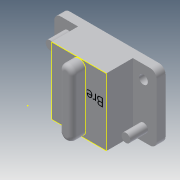
# Autodesk Inventor part: circuit breaker
Saved by Autodesk Inventor 2014 (Build 180170000, 170)
## iProperties
Created: 2016-01-13
Part Number: circuit breaker
Material: Generic
Document SubType Name: Modeling
Designer: Paul
Density: 1 g/cm^3
Appearance: Default
Author: Paul
Autodesk Inventor part; units mm, degrees
ref_plane "YZ Plane" through (0, 0, 0) normal (1, 0, 0) x (0, 1, 0)
ref_plane "XZ Plane" through (0, 0, 0) normal (0, 1, 0) x (-1, 0, 0)
ref_plane "XY Plane" through (0, 0, 0) normal (0, 0, 1) x (1, 0, 0)
sketch "Sketch1" plane through (0, 0, 0) normal (0, 0, 1) x (1, 0, 0)
  line L0 (4.7625, 0) -> (68.8975, 0)
  line L1 (73.66, 4.7625) -> (73.66, 43.4975)
  line L2 (68.8975, 48.26) -> (4.7625, 48.26)
  line L3 (0, 43.4975) -> (0, 4.7625)
  arc A0 (0, 4.7625) -> (4.7625, 0) centre (4.7625, 4.7625) ccw
  arc A1 (4.7625, 48.26) -> (0, 43.4975) centre (4.7625, 43.4975) ccw
  arc A2 (73.66, 43.4975) -> (68.8975, 48.26) centre (68.8975, 43.4975) ccw
  arc A3 (68.8975, 0) -> (73.66, 4.7625) centre (68.8975, 4.7625) ccw
  circle A4 centre (9.525, 9.525) radius 3.175
  circle A5 centre (64.135, 38.735) radius 3.175
  point P0 (0, 0)
  point P1 (73.66, 48.26)
  point P2 (73.66, 0)
  point P3 (0, 48.26)
  dimension "d0" = 73.66
  dimension "d1" = 48.26
  dimension "d2" = 4.7625
  dimension "d3" = 6.35
  dimension "d4" = 6.35
  dimension "d15" = 9.525
  dimension "d16" = 9.525
  dimension "d17" = 9.525
  dimension "d18" = 9.525
  constraints: 8 end point, 8 point on circle, 8 point on line, 8 tangent, 6 centre point, 3 equal radius, 2 parallel, 1 horizontal, 1 perpendicular
  measures "d0" distance of point (0, 48.26) point (73.66, 48.26)
  measures "d1" distance of point (73.66, 48.26) point (73.66, 0)
  measures "d2" radius of A0
  measures "d3" diameter of A4
  measures "d4" diameter of A5
  measures "d15" distance from line of A4.centre L3
  measures "d16" distance from line of A4.centre L0
  measures "d17" distance from line of L1 A5.centre
  measures "d18" distance from line of A5.centre L2
extrude "Extrusion1" add sketch "Sketch1" along normal blind 6.35
sketch "Sketch2" plane through (0, 0, 6.35) normal (0, 0, 1) x (1, 0, 0)
  line L0 (4.7625, 0) -> (68.8975, 0) projected
  line L1 (68.8975, 48.26) -> (4.7625, 48.26) projected
  line L2 (17.145, 48.26) -> (56.515, 48.26)
  line L3 (56.515, 48.26) -> (56.515, 0)
  line L4 (56.515, 0) -> (17.145, 0)
  line L5 (17.145, 0) -> (17.145, 48.26)
  point P0 (0, 0)
  point P1 (36.83, 48.26)
  dimension "d7" = 39.37
  constraints: 8 end point, 2 midpoint, 2 parallel, 2 point on line, 1 horizontal, 1 perpendicular
  measures "d7" distance between parallel lines of L5 L3
extrude "Extrusion2" add sketch "Sketch2" along normal blind 19.05
sketch "Sketch3" plane through (0, 0, 25.4) normal (0, 0, 1) x (1, 0, 0)
  line L0 (56.515, 0) -> (56.515, 48.26) projected
  line L1 (36.83, 43.0529) -> (36.83, 5.2071) construction
  line L2 (31.9271, 43.0529) -> (31.9271, 5.2071)
  line L3 (41.7329, 5.2071) -> (41.7329, 43.0529)
  arc A0 (41.7329, 43.0529) -> (31.9271, 43.0529) centre (36.83, 43.0529) ccw
  arc A1 (31.9271, 5.2071) -> (41.7329, 5.2071) centre (36.83, 5.2071) ccw
  point P0 (0, 0)
  point P1 (36.83, 24.13)
  constraints: 8 end point, 4 point on circle, 4 tangent, 2 centre point, 2 parallel, 1 midpoint
extrude "Extrusion3" add sketch "Sketch3" along normal blind 9.525
fillet "Fillet1" radius 3.175 4 edges at (36.83, 47.9557, 34.925) (31.9271, 24.13, 34.925) (36.83, 0.3043, 34.925) (41.7329, 24.13, 34.925)
sketch "Sketch4" plane through (0, 0, 6.35) normal (0, 0, 1) x (1, 0, 0)
  line L0 (17.145, 0) -> (17.145, 48.26) projected
  line L1 (17.145, 48.26) -> (4.7625, 48.26) projected
  arc A0 (4.7625, 48.26) -> (0, 43.4975) centre (4.7625, 43.4975) ccw projected
  line L2 (0, 43.4975) -> (0, 4.7625) projected
  arc A1 (0, 4.7625) -> (4.7625, 0) centre (4.7625, 4.7625) ccw projected
  line L3 (4.7625, 0) -> (17.145, 0) projected
  circle A2 centre (9.525, 9.525) radius 3.175 projected
  circle A3 centre (9.7398, 39.2035) radius 3.175
  circle A4 centre (64.2147, 8.8123) radius 3.175
  point P0 (0, 0)
  constraints: 2 centre point
extrude "Extrusion4" add sketch "Sketch4" along normal blind 12.7 contours A3 | A4
sketch "Sketch5" plane through (0, 0, 25.4) normal (0, 0, 1) x (1, 0, 0)
  arc A0 (41.7329, 43.0529) -> (31.9271, 43.0529) centre (36.83, 43.0529) ccw projected
  line L0 (41.7329, 43.0529) -> (41.7329, 5.2071) projected
  arc A1 (31.9271, 5.2071) -> (41.7329, 5.2071) centre (36.83, 5.2071) ccw projected
  line L1 (31.9271, 5.2071) -> (31.9271, 43.0529) projected
  line L2 (56.515, 0) -> (56.515, 48.26) projected
  line L3 (56.515, 48.26) -> (17.145, 48.26) projected
  line L4 (17.145, 48.26) -> (17.145, 0) projected
  line L5 (17.145, 0) -> (56.515, 0) projected
  line L6 (54.6348, 25.4202) -> (38.8658, 25.4202) construction
  line L7 (38.8658, 25.4202) -> (38.8658, -8.6983) construction
  line L8 (38.8658, -8.6983) -> (54.6348, -8.6983) construction
  line L9 (54.6348, -8.6983) -> (54.6348, 25.4202) construction
  point P0 (0, 0)
  constraints: 2 other
body "Solid1"
